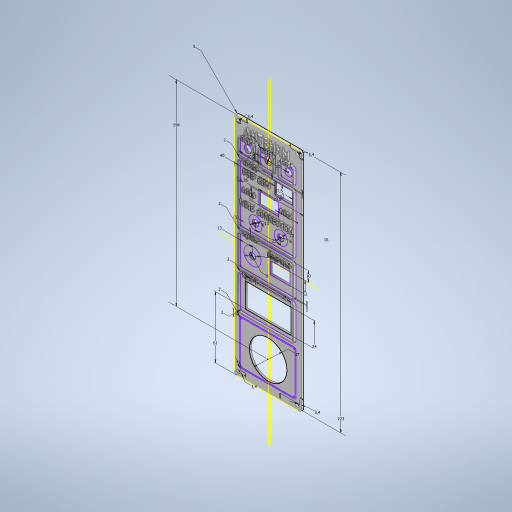
# Autodesk Inventor part: блок ЗИП и портов
Saved by Autodesk Inventor 2023.1 (Build 271208000, 208)
## iProperties
Created: 2023-03-03
Part Number: блок ЗИП и портов
Material: Типовые
Document SubType Name: Modeling
Designer: User
Density: 1 g/cm^3
Appearance: По умолчанию
Author: User
Autodesk Inventor part; units mm, degrees
(part 1 of 3)
ref_plane "YZ Plane" through (0, 0, 0) normal (1, 0, 0) x (0, 1, 0)
ref_plane "XZ Plane" through (0, 0, 0) normal (0, 1, 0) x (-1, 0, 0)
ref_plane "XY Plane" through (0, 0, 0) normal (0, 0, 1) x (1, 0, 0)
sketch "Эскиз1" plane through (0, 0, 0) normal (0, 0, 1) x (1, 0, 0)
  line L0 (-30.175, 111.5) -> (30.175, 111.5)
  line L1 (33.175, 108.5) -> (33.175, -108.5)
  line L2 (30.175, -111.5) -> (-30.175, -111.5)
  line L3 (-33.175, -108.5) -> (-33.175, 108.5)
  line L4 (0, -156.9698) -> (0, 156.9698) projected
  line L5 (-47.3148, 0) -> (47.3148, 0) projected
  arc A0 (-30.175, 111.5) -> (-33.175, 108.5) centre (-30.175, 108.5) ccw
  arc A1 (33.175, 108.5) -> (30.175, 111.5) centre (30.175, 108.5) ccw
  arc A2 (-33.175, -108.5) -> (-30.175, -111.5) centre (-30.175, -108.5) ccw
  arc A3 (30.175, -111.5) -> (33.175, -108.5) centre (30.175, -108.5) ccw
  circle A4 centre (-29.175, 107.5) radius 1.7
  circle A5 centre (29.175, 107.5) radius 1.7
  circle A6 centre (-29.175, -107.5) radius 1.7
  circle A7 centre (29.175, -107.5) radius 1.7
  point P0 (0, 0)
  dimension "d0" = 223
  dimension "d1" = 66.35
  dimension "d2" = 3
  dimension "d3" = 3.4
  dimension "d4" = 3.4
  dimension "d5" = 3.4
  dimension "d6" = 3.4
  dimension "d7" = 4
  dimension "d8" = 4
  dimension "d9" = 4
  dimension "d10" = 4
  dimension "d11" = 4
  dimension "d12" = 4
  dimension "d13" = 4
  dimension "d14" = 4
  constraints: 8 centre point, 8 end point, 8 point on circle, 8 tangent, 3 equal radius, 2 parallel, 1 horizontal, 1 perpendicular, 2 other
  measures "d0" distance between parallel lines of L2 L0
  measures "d1" distance between parallel lines of L3 L1
  measures "d2" radius of A0
  measures "d3" diameter of A4
  measures "d4" diameter of A5
  measures "d5" diameter of A6
  measures "d6" diameter of A7
  measures "d7" distance from line of L3 A6.centre
  measures "d8" distance from line of L2 A6.centre
  measures "d9" distance from line of L2 A7.centre
  measures "d10" distance from line of L1 A7.centre
  measures "d11" distance from line of A4.centre L0
  measures "d12" distance from line of L3 A4.centre
  measures "d13" distance from line of L0 A5.centre
  measures "d14" distance from line of L1 A5.centre
extrude "Выдавливание1" add sketch "Эскиз1" along normal blind 2
sketch "Эскиз2" plane through (0, 0, 2) normal (0, 0, 1) x (1, 0, 0)
  line L0 (-23.4853, 106.5513) -> (31.3754, 106.5513) construction
  line L1 (31.3754, 106.5513) -> (31.3754, 99.1453) construction
  line L2 (31.3754, 99.1453) -> (-23.4853, 99.1453) construction
  line L3 (-23.4853, 99.1453) -> (-23.4853, 106.5513) construction
  circle A0 centre (0, 87.4719) radius 3.5
  line L4 (6.5101, 93.4723) -> (6.5101, 81.4719)
  line L5 (5.5101, 80.4719) -> (-6.4899, 80.4719)
  line L6 (-7.4899, 81.4719) -> (-7.4899, 93.4723)
  arc A1 (-6.4899, 94.4723) -> (-7.4899, 93.4723) centre (-6.4899, 93.4723) ccw
  arc A2 (6.5101, 93.4723) -> (5.5101, 94.4723) centre (5.5101, 93.4723) ccw
  arc A3 (5.5101, 80.4719) -> (6.5101, 81.4719) centre (5.5101, 81.4719) ccw
  arc A4 (-7.4899, 81.4719) -> (-6.4899, 80.4719) centre (-6.4899, 81.4719) ccw
  line L7 (-8.4899, 93.4723) -> (-8.4899, 81.4719)
  arc A5 (-8.4899, 81.4719) -> (-6.4899, 79.4719) centre (-6.4899, 81.4719) ccw
  line L8 (-6.4899, 79.4719) -> (5.5101, 79.4719)
  arc A6 (5.5101, 79.4719) -> (7.5101, 81.4719) centre (5.5101, 81.4719) ccw
  line L9 (7.5101, 81.4719) -> (7.5101, 93.4723)
  arc A7 (7.5101, 93.4723) -> (5.5101, 95.4723) centre (5.5101, 93.4723) ccw
  arc A8 (-6.4899, 95.4723) -> (-8.4899, 93.4723) centre (-6.4899, 93.4723) ccw
  line L10 (-6.4899, 94.4723) -> (-6.4899, 95.4723)
  line L11 (-5.4694, 97.1945) -> (11.2685, 97.1945) construction
  line L12 (11.2685, 97.1945) -> (11.2685, 90.8671) construction
  line L13 (11.2685, 90.8671) -> (-5.4694, 90.8671) construction
  line L14 (-5.4694, 90.8671) -> (-5.4694, 97.1945) construction
  line L15 (5.5101, 94.4723) -> (5.5101, 95.4723)
  circle A9 centre (20, 87.4719) radius 3.5
  line L16 (26.5101, 93.4723) -> (26.5101, 81.4719)
  line L17 (25.5101, 80.4719) -> (13.5101, 80.4719)
  line L18 (13.5101, 79.4719) -> (25.5101, 79.4719)
  arc A10 (26.5101, 93.4723) -> (25.5101, 94.4723) centre (25.5101, 93.4723) ccw
  line L19 (27.5101, 81.4719) -> (27.5101, 93.4723)
  line L20 (25.5101, 94.4723) -> (25.5101, 95.4723)
  arc A11 (27.5101, 93.4723) -> (25.5101, 95.4723) centre (25.5101, 93.4723) ccw
  arc A12 (25.5101, 80.4719) -> (26.5101, 81.4719) centre (25.5101, 81.4719) ccw
  arc A13 (25.5101, 79.4719) -> (27.5101, 81.4719) centre (25.5101, 81.4719) ccw
  arc A14 (13.5101, 94.4723) -> (12.5101, 93.4723) centre (13.5101, 93.4723) ccw
  line L21 (13.5101, 94.4723) -> (13.5101, 95.4723)
  arc A15 (13.5101, 95.4723) -> (11.5101, 93.4723) centre (13.5101, 93.4723) ccw
  arc A16 (11.5101, 81.4719) -> (13.5101, 79.4719) centre (13.5101, 81.4719) ccw
  line L22 (12.5101, 81.4719) -> (12.5101, 93.4723)
  line L23 (11.5101, 93.4723) -> (11.5101, 81.4719)
  arc A17 (12.5101, 81.4719) -> (13.5101, 80.4719) centre (13.5101, 81.4719) ccw
  line L24 (13.4684, 97.2035) -> (30.2064, 97.2035) construction
  line L25 (30.2064, 97.2035) -> (30.2064, 90.8761) construction
  line L26 (30.2064, 90.8761) -> (13.4684, 90.8761) construction
  line L27 (13.4684, 90.8761) -> (13.4684, 97.2035) construction
  arc A18 (-28.4899, 81.4719) -> (-26.4899, 79.4719) centre (-26.4899, 81.4719) ccw
  line L28 (-12.4899, 81.4719) -> (-12.4899, 93.4723)
  arc A19 (-27.4899, 81.4719) -> (-26.4899, 80.4719) centre (-26.4899, 81.4719) ccw
  line L29 (-26.4899, 79.4719) -> (-14.4899, 79.4719)
  line L30 (-27.4899, 81.4719) -> (-27.4899, 93.4723)
  line L31 (-28.4899, 93.4723) -> (-28.4899, 81.4719)
  arc A20 (-26.4899, 95.4723) -> (-28.4899, 93.4723) centre (-26.4899, 93.4723) ccw
  arc A21 (-26.4899, 94.4723) -> (-27.4899, 93.4723) centre (-26.4899, 93.4723) ccw
  line L32 (-14.4899, 80.4719) -> (-26.4899, 80.4719)
  arc A22 (-14.4899, 80.4719) -> (-13.4899, 81.4719) centre (-14.4899, 81.4719) ccw
  line L33 (-26.4899, 94.4723) -> (-26.4899, 95.4723)
  circle A23 centre (-20, 87.4719) radius 3.5
  line L34 (-13.4899, 93.4723) -> (-13.4899, 81.4719)
  arc A24 (-13.4899, 93.4723) -> (-14.4899, 94.4723) centre (-14.4899, 93.4723) ccw
  line L35 (-14.4899, 94.4723) -> (-14.4899, 95.4723)
  arc A25 (-12.4899, 93.4723) -> (-14.4899, 95.4723) centre (-14.4899, 93.4723) ccw
  arc A26 (-14.4899, 79.4719) -> (-12.4899, 81.4719) centre (-14.4899, 81.4719) ccw
  line L36 (-25.5636, 97.0542) -> (-8.8256, 97.0542) construction
  line L37 (-8.8256, 97.0542) -> (-8.8256, 90.7268) construction
  line L38 (-8.8256, 90.7268) -> (-25.5636, 90.7268) construction
  line L39 (-25.5636, 90.7268) -> (-25.5636, 97.0542) construction
  line L40 (6.825, 73.4719) -> (24.325, 73.4719)
  line L41 (24.325, 73.4719) -> (24.325, 61.4719)
  line L42 (24.325, 61.4719) -> (6.825, 61.4719)
  line L43 (6.825, 61.4719) -> (6.825, 73.4719)
  line L44 (0, -156.1) -> (0, 156.1) projected
  line L45 (-23.9479, 69.9979) -> (9.951, 69.9979) construction
  line L46 (9.951, 69.9979) -> (9.951, 63.8878) construction
  line L47 (9.951, 63.8878) -> (-23.9479, 63.8878) construction
  line L48 (-23.9479, 63.8878) -> (-23.9479, 69.9979) construction
  line L49 (-33.175, 108.5) -> (-33.175, -108.5) projected
  line L50 (27.5101, 74.3869) -> (27.5101, 19.3056)
  line L51 (25.5101, 17.3056) -> (-26.4899, 17.3056)
  line L52 (-28.4899, 19.3056) -> (-28.4899, 74.3869)
  arc A27 (-26.4899, 76.3869) -> (-28.4899, 74.3869) centre (-26.4899, 74.3869) ccw
  arc A28 (27.5101, 74.3869) -> (25.5101, 76.3869) centre (25.5101, 74.3869) ccw
  arc A29 (25.5101, 17.3056) -> (27.5101, 19.3056) centre (25.5101, 19.3056) ccw
  arc A30 (-28.4899, 19.3056) -> (-26.4899, 17.3056) centre (-26.4899, 19.3056) ccw
  arc A31 (-26.4899, 75.3869) -> (-27.4899, 74.3869) centre (-26.4899, 74.3869) ccw
  line L53 (-27.4899, 74.3869) -> (-27.4899, 19.3056)
  arc A32 (-27.4899, 19.3056) -> (-26.4899, 18.3056) centre (-26.4899, 19.3056) ccw
  line L54 (-26.4899, 18.3056) -> (25.5101, 18.3056)
  arc A33 (25.5101, 18.3056) -> (26.5101, 19.3056) centre (25.5101, 19.3056) ccw
  line L55 (26.5101, 19.3056) -> (26.5101, 74.3869)
  arc A34 (26.5101, 74.3869) -> (25.5101, 75.3869) centre (25.5101, 74.3869) ccw
  line L56 (-24.4499, 53.724) -> (9.4489, 53.724) construction
  line L57 (9.4489, 53.724) -> (9.4489, 47.6139) construction
  line L58 (9.4489, 47.6139) -> (-24.4499, 47.6139) construction
  line L59 (-24.4499, 47.6139) -> (-24.4499, 53.724) construction
  line L60 (-8.9899, 57.0024) -> (10.5101, 57.0024)
  line L61 (10.5101, 57.0024) -> (10.5101, 45.0024)
  line L62 (10.5101, 45.0024) -> (-8.9899, 45.0024)
  line L63 (-8.9899, 45.0024) -> (-8.9899, 57.0024)
  line L64 (12.474, 47.646) -> (12.474, 53.7562) construction
  line L65 (12.474, 53.7562) -> (46.3728, 53.7562) construction
  line L66 (46.3728, 53.7562) -> (46.3728, 47.646) construction
  line L67 (46.3728, 47.646) -> (12.474, 47.646) construction
  line L68 (-27.2571, 42.4637) -> (29.1197, 42.4637) construction
  line L69 (29.1197, 42.4637) -> (29.1197, 45.205) construction
  line L70 (29.1197, 45.205) -> (-27.2571, 45.205) construction
  line L71 (-27.2571, 45.205) -> (-27.2571, 42.4637) construction
  circle A35 centre (-12.5, 27.8557) radius 3
  circle A36 centre (12.5, 27.8557) radius 3
  circle A37 centre (-12.5, 27.8557) radius 6.5
  circle A38 centre (12.5, 27.8557) radius 6.5
  line L72 (-24.9853, 76.3869) -> (-24.9853, 75.3869)
  line L73 (-26.4899, 76.3869) -> (-24.9853, 76.3869)
  line L74 (-6.4899, 76.3869) -> (25.5101, 76.3869)
  line L75 (-24.9853, 75.3869) -> (-26.4899, 75.3869)
  line L76 (-23.3758, 71.3083) -> (-23.3758, 77.6357) construction
  line L77 (-23.3758, 77.6357) -> (-6.6378, 77.6357) construction
  line L78 (-6.6378, 77.6357) -> (-6.6378, 71.3083) construction
  line L79 (-6.6378, 71.3083) -> (-23.3758, 71.3083) construction
  line L80 (-6.4899, 76.3869) -> (-6.4899, 75.3869)
  line L81 (25.5101, 75.3869) -> (-6.4899, 75.3869)
  line L82 (-12.4899, 74.9766) -> (-12.5, 74.9766)
  line L83 (27.5101, 12.3056) -> (27.5101, -15.7398)
  line L84 (25.5101, -17.7398) -> (-26.4899, -17.7398)
  line L85 (-28.4899, -15.7398) -> (-28.4899, 12.3056)
  arc A39 (-26.4899, 14.3056) -> (-28.4899, 12.3056) centre (-26.4899, 12.3056) ccw
  arc A40 (-28.4899, -15.7398) -> (-26.4899, -17.7398) centre (-26.4899, -15.7398) ccw
  arc A41 (25.5101, -17.7398) -> (27.5101, -15.7398) centre (25.5101, -15.7398) ccw
  arc A42 (27.5101, 12.3056) -> (25.5101, 14.3056) centre (25.5101, 12.3056) ccw
  arc A43 (-26.4899, 13.3056) -> (-27.4899, 12.3056) centre (-26.4899, 12.3056) ccw
  line L86 (-27.4899, 12.3056) -> (-27.4899, -15.7398)
  arc A44 (-27.4899, -15.7398) -> (-26.4899, -16.7398) centre (-26.4899, -15.7398) ccw
  line L87 (-26.4899, -16.7398) -> (25.5101, -16.7398)
  arc A45 (25.5101, -16.7398) -> (26.5101, -15.7398) centre (25.5101, -15.7398) ccw
  line L88 (26.5101, -15.7398) -> (26.5101, 12.3056)
  arc A46 (26.5101, 12.3056) -> (25.5101, 13.3056) centre (25.5101, 12.3056) ccw
  line L89 (-24.4499, 14.3056) -> (-24.4499, 13.3056)
  line L90 (-26.4899, 14.3056) -> (-24.4499, 14.3056)
  line L91 (-8.4899, 14.3056) -> (25.5101, 14.3056)
  line L92 (25.5101, 13.3056) -> (-8.4899, 13.3056)
  line L93 (-24.4499, 13.3056) -> (-26.4899, 13.3056)
  line L94 (-23.3782, 9.1957) -> (-23.3782, 15.5231) construction
  line L95 (-23.3782, 15.5231) -> (-6.6403, 15.5231) construction
  line L96 (-6.6403, 15.5231) -> (-6.6403, 9.1957) construction
  line L97 (-6.6403, 9.1957) -> (-23.3782, 9.1957) construction
  line L98 (-8.4899, 14.3056) -> (-8.4899, 13.3056)
  circle A47 centre (-15.4899, -1.7171) radius 3
  circle A48 centre (-15.4899, -1.7171) radius 8.5
  line L99 (2.2026, 3.3056) -> (21.7026, 3.3056)
  line L100 (21.7026, 3.3056) -> (21.7026, -8.6944)
  line L101 (21.7026, -8.6944) -> (2.2026, -8.6944)
  line L102 (2.2026, -8.6944) -> (2.2026, 3.3056)
  line L103 (0.6713, 5.0746) -> (0.6713, 11.009) construction
  line L104 (0.6713, 11.009) -> (17.4092, 11.009) construction
  line L105 (17.4092, 11.009) -> (17.4092, 5.0746) construction
  line L106 (17.4092, 5.0746) -> (0.6713, 5.0746) construction
  line L107 (27.5101, -22.4503) -> (27.5101, -52.9823)
  line L108 (25.5101, -54.9823) -> (-26.4899, -54.9823)
  line L109 (-28.4899, -52.9823) -> (-28.4899, -22.4503)
  arc A49 (-26.4899, -20.4503) -> (-28.4899, -22.4503) centre (-26.4899, -22.4503) ccw
  arc A50 (-28.4899, -52.9823) -> (-26.4899, -54.9823) centre (-26.4899, -52.9823) ccw
  arc A51 (25.5101, -54.9823) -> (27.5101, -52.9823) centre (25.5101, -52.9823) ccw
  arc A52 (27.5101, -22.4503) -> (25.5101, -20.4503) centre (25.5101, -22.4503) ccw
  arc A53 (-26.4899, -21.4503) -> (-27.4899, -22.4503) centre (-26.4899, -22.4503) ccw
  line L110 (-27.4899, -22.4503) -> (-27.4899, -52.9823)
  arc A54 (-27.4899, -52.9823) -> (-26.4899, -53.9823) centre (-26.4899, -52.9823) ccw
  line L111 (-26.4899, -53.9823) -> (25.5101, -53.9823)
  arc A55 (25.5101, -53.9823) -> (26.5101, -52.9823) centre (25.5101, -52.9823) ccw
  line L112 (26.5101, -52.9823) -> (26.5101, -22.4503)
  arc A56 (26.5101, -22.4503) -> (25.5101, -21.4503) centre (25.5101, -22.4503) ccw
  line L113 (-22.5, -26.5) -> (22.5, -26.5)
  line L114 (22.5, -26.5) -> (22.5, -50.5)
  line L115 (22.5, -50.5) -> (-22.5, -50.5)
  line L116 (-22.5, -50.5) -> (-22.5, -26.5)
  line L117 (-30.175, -111.5) -> (30.175, -111.5) projected
  line L118 (-25.4699, -20.4503) -> (-25.4699, -21.4503)
  line L119 (-8.4899, -20.4503) -> (-8.4899, -21.4503)
  line L120 (25.5101, -21.4503) -> (-8.4899, -21.4503)
  line L121 (-25.4699, -21.4503) -> (-26.4899, -21.4503)
  line L122 (-26.4899, -20.4503) -> (-25.4699, -20.4503)
  line L123 (-8.4899, -20.4503) -> (25.5101, -20.4503)
  line L124 (-23.7978, -25.6666) -> (-23.7978, -19.3393) construction
  line L125 (-23.7978, -19.3393) -> (-7.0599, -19.3393) construction
  line L126 (-7.0599, -19.3393) -> (-7.0599, -25.6666) construction
  line L127 (-7.0599, -25.6666) -> (-23.7978, -25.6666) construction
  circle A57 centre (0, -82.5) radius 18.5
  line L128 (30.175, 111.5) -> (-30.175, 111.5) projected
  line L129 (-26.4899, -58.9749) -> (25.5101, -58.9749)
  line L130 (27.5101, -60.9749) -> (27.5101, -101.3327)
  line L131 (25.5101, -103.3327) -> (-26.4899, -103.3327)
  line L132 (-28.4899, -101.3327) -> (-28.4899, -60.9749)
  arc A58 (-26.4899, -58.9749) -> (-28.4899, -60.9749) centre (-26.4899, -60.9749) ccw
  arc A59 (27.5101, -60.9749) -> (25.5101, -58.9749) centre (25.5101, -60.9749) ccw
  arc A60 (25.5101, -103.3327) -> (27.5101, -101.3327) centre (25.5101, -101.3327) ccw
  arc A61 (-28.4899, -101.3327) -> (-26.4899, -103.3327) centre (-26.4899, -101.3327) ccw
  line L133 (25.5101, -59.9749) -> (-26.4899, -59.9749)
  arc A62 (-26.4899, -59.9749) -> (-27.4899, -60.9749) centre (-26.4899, -60.9749) ccw
  line L134 (-27.4899, -60.9749) -> (-27.4899, -101.3327)
  arc A63 (-27.4899, -101.3327) -> (-26.4899, -102.3327) centre (-26.4899, -101.3327) ccw
  line L135 (-26.4899, -102.3327) -> (25.5101, -102.3327)
  arc A64 (25.5101, -102.3327) -> (26.5101, -101.3327) centre (25.5101, -101.3327) ccw
  line L136 (26.5101, -101.3327) -> (26.5101, -60.9749)
  arc A65 (26.5101, -60.9749) -> (25.5101, -59.9749) centre (25.5101, -60.9749) ccw
  line L137 (-23.2368, 95.4767) -> (-23.2368, 96.7836)
  spline S0 degree 2 poles (-23.2368, 96.7836) (-23.2368, 97.0344) (-22.986, 97.0344) knots 0 0 0 1 1 1
  spline S1 degree 2 poles (-22.986, 97.0344) (-22.7352, 97.0344) (-22.7352, 96.7836) knots 0 0 0 1 1 1
  line L138 (-22.7352, 96.7836) -> (-22.7352, 93.2985)
  spline S2 degree 2 poles (-22.7352, 93.2985) (-22.7352, 93.0443) (-22.9926, 93.0443) knots 0 0 0 1 1 1
  spline S3 degree 2 poles (-22.9926, 93.0443) (-23.2368, 93.0443) (-23.2368, 93.2919) knots 0 0 0 1 1 1
  line L139 (-23.2368, 93.2919) -> (-23.2368, 94.9783)
  line L140 (-23.2368, 94.9783) -> (-24.6758, 94.9783)
  line L141 (-24.6758, 94.9783) -> (-24.6758, 93.2919)
  spline S4 degree 2 poles (-24.6758, 93.2919) (-24.6758, 93.041) (-24.9266, 93.041) knots 0 0 0 1 1 1
  spline S5 degree 2 poles (-24.9266, 93.041) (-25.1774, 93.041) (-25.1774, 93.2919) knots 0 0 0 1 1 1
  line L142 (-25.1774, 93.2919) -> (-25.1774, 96.777)
  spline S6 degree 2 poles (-25.1774, 96.777) (-25.1774, 97.0278) (-24.9266, 97.0278) knots 0 0 0 1 1 1
  spline S7 degree 2 poles (-24.9266, 97.0278) (-24.6758, 97.0278) (-24.6758, 96.777) knots 0 0 0 1 1 1
  line L143 (-24.6758, 96.777) -> (-24.6758, 95.4767)
  line L144 (-24.6758, 95.4767) -> (-23.2368, 95.4767)
  line L145 (-20.2731, 93.041) -> (-21.0487, 93.041)
  spline S8 degree 2 poles (-21.0487, 93.041) (-21.4745, 93.041) (-22.0718, 93.6384) (-22.0718, 94.0674) knots 0 0 0 1 2 2 2
  line L146 (-22.0718, 94.0674) -> (-22.0718, 96.0047)
  spline S9 degree 2 poles (-22.0718, 96.0047) (-22.0718, 96.4305) (-21.4745, 97.0278) (-21.0487, 97.0278) knots 0 0 0 1 2 2 2
  line L147 (-21.0487, 97.0278) -> (-20.2731, 97.0278)
  spline S10 degree 2 poles (-20.2731, 97.0278) (-20.019, 97.0278) (-20.019, 96.7803) knots 0 0 0 1 1 1
  spline S11 degree 2 poles (-20.019, 96.7803) (-20.019, 96.5295) (-20.2731, 96.5295) knots 0 0 0 1 1 1
  line L148 (-20.2731, 96.5295) -> (-21.0487, 96.5295)
  spline S12 degree 2 poles (-21.0487, 96.5295) (-21.2632, 96.5295) (-21.5702, 96.2226) (-21.5702, 96.0047) knots 0 0 0 1 2 2 2
  line L149 (-21.5702, 96.0047) -> (-21.5702, 94.0641)
  spline S13 degree 2 poles (-21.5702, 94.0641) (-21.5702, 93.8463) (-21.2632, 93.5394) (-21.0487, 93.5394) knots 0 0 0 1 2 2 2
  line L150 (-21.0487, 93.5394) -> (-20.2731, 93.5394)
  spline S14 degree 2 poles (-20.2731, 93.5394) (-20.019, 93.5394) (-20.019, 93.2919) knots 0 0 0 1 1 1
  spline S15 degree 2 poles (-20.019, 93.2919) (-20.019, 93.041) (-20.2731, 93.041) knots 0 0 0 1 1 1
  spline S16 degree 2 poles (-18.0817, 93.2919) (-18.0817, 93.041) (-18.3325, 93.041) knots 0 0 0 1 1 1
  spline S17 degree 2 poles (-18.3325, 93.041) (-18.5834, 93.041) (-18.5834, 93.2886) knots 0 0 0 1 1 1
  line L151 (-18.5834, 93.2886) -> (-18.5834, 96.2556)
  line L152 (-18.5834, 96.2556) -> (-18.9332, 95.8265)
  spline S18 degree 2 poles (-18.9332, 95.8265) (-19.0058, 95.7539) (-19.1048, 95.7539) knots 0 0 0 1 1 1
  spline S19 degree 2 poles (-19.1048, 95.7539) (-19.2071, 95.7539) (-19.3589, 95.9057) (-19.3589, 96.008) knots 0 0 0 1 2 2 2
  spline S20 degree 2 poles (-19.3589, 96.008) (-19.3589, 96.1037) (-19.2863, 96.1763) knots 0 0 0 1 1 1
  line L153 (-19.2863, 96.1763) -> (-18.5108, 96.9519)
  spline S21 degree 2 poles (-18.5108, 96.9519) (-18.4084, 97.0542) (-18.2995, 97.0542) knots 0 0 0 1 1 1
  spline S22 degree 2 poles (-18.2995, 97.0542) (-18.0817, 97.0542) (-18.0817, 96.777) knots 0 0 0 1 1 1
  line L154 (-18.0817, 96.777) -> (-18.0817, 93.2919)
  line L155 (-15.5075, 95.4833) -> (-16.7616, 93.5394)
  line L156 (-16.7616, 93.5394) -> (-15.6197, 93.5394)
  spline S23 degree 2 poles (-15.6197, 93.5394) (-15.3655, 93.5394) (-15.3655, 93.2919) knots 0 0 0 1 1 1
  spline S24 degree 2 poles (-15.3655, 93.2919) (-15.3655, 93.041) (-15.6197, 93.041) knots 0 0 0 1 1 1
  line L157 (-15.6197, 93.041) -> (-17.1708, 93.041)
  spline S25 degree 2 poles (-17.1708, 93.041) (-17.4348, 93.041) (-17.4348, 93.2523) knots 0 0 0 1 1 1
  spline S26 degree 2 poles (-17.4348, 93.2523) (-17.4348, 93.3315) (-17.3688, 93.4437) knots 0 0 0 1 1 1
  line L158 (-17.3688, 93.4437) -> (-15.9497, 95.7044)
  spline S27 degree 2 poles (-15.9497, 95.7044) (-15.8738, 95.8298) (-15.8738, 95.9717) knots 0 0 0 1 1 1
  spline S28 degree 2 poles (-15.8738, 95.9717) (-15.8738, 96.1895) (-16.2137, 96.5262) (-16.4579, 96.5262) knots 0 0 0 1 2 2 2
  spline S29 degree 2 poles (-16.4579, 96.5262) (-16.7814, 96.5262) (-16.9563, 96.2523) knots 0 0 0 1 1 1
  spline S30 degree 2 poles (-16.9563, 96.2523) (-17.0322, 96.14) (-17.1609, 96.14) knots 0 0 0 1 1 1
  spline S31 degree 2 poles (-17.1609, 96.14) (-17.2665, 96.14) (-17.4249, 96.282) (-17.4249, 96.3876) knots 0 0 0 1 2 2 2
  spline S32 degree 2 poles (-17.4249, 96.3876) (-17.4249, 96.4602) (-17.3754, 96.5328) knots 0 0 0 1 1 1
  spline S33 degree 2 poles (-17.3754, 96.5328) (-17.0487, 97.0311) (-16.4579, 97.0311) knots 0 0 0 1 1 1
  spline S34 degree 2 poles (-16.4579, 97.0311) (-16.0058, 97.0311) (-15.3655, 96.3843) (-15.3655, 95.9651) knots 0 0 0 1 2 2 2
  spline S35 degree 2 poles (-15.3655, 95.9651) (-15.3655, 95.6879) (-15.5075, 95.4833) knots 0 0 0 1 1 1
  spline S36 degree 2 poles (-20.4591, 66.2427) (-20.4591, 65.7265) (-21.1877, 64.9979) (-21.7039, 64.9979) knots 0 0 0 1 2 2 2
  line L159 (-21.7039, 64.9979) -> (-22.2035, 64.9979)
  spline S37 degree 2 poles (-22.2035, 64.9979) (-22.7197, 64.9979) (-23.4483, 65.7265) (-23.4483, 66.2427) knots 0 0 0 1 2 2 2
  line L160 (-23.4483, 66.2427) -> (-23.4483, 69.7315)
  spline S38 degree 2 poles (-23.4483, 69.7315) (-23.4483, 69.9813) (-23.1985, 69.9813) knots 0 0 0 1 1 1
  spline S39 degree 2 poles (-23.1985, 69.9813) (-22.9487, 69.9813) (-22.9487, 69.7315) knots 0 0 0 1 1 1
  line L161 (-22.9487, 69.7315) -> (-22.9487, 66.2469)
  spline S40 degree 2 poles (-22.9487, 66.2469) (-22.9487, 65.9346) (-22.5116, 65.4975) (-22.2035, 65.4975) knots 0 0 0 1 2 2 2
  line L162 (-22.2035, 65.4975) -> (-21.7039, 65.4975)
  spline S41 degree 2 poles (-21.7039, 65.4975) (-21.3958, 65.4975) (-20.9587, 65.9346) (-20.9587, 66.2469) knots 0 0 0 1 2 2 2
  line L163 (-20.9587, 66.2469) -> (-20.9587, 69.7315)
  spline S42 degree 2 poles (-20.9587, 69.7315) (-20.9587, 69.9813) (-20.7089, 69.9813) knots 0 0 0 1 1 1
  spline S43 degree 2 poles (-20.7089, 69.9813) (-20.4591, 69.9813) (-20.4591, 69.7315) knots 0 0 0 1 1 1
  line L164 (-20.4591, 69.7315) -> (-20.4591, 66.2427)
  spline S44 degree 2 poles (-16.6248, 69.5608) (-16.5124, 69.4817) (-16.5124, 69.361) knots 0 0 0 1 1 1
  spline S45 degree 2 poles (-16.5124, 69.361) (-16.5124, 69.261) (-16.6623, 69.1028) (-16.7622, 69.1028) knots 0 0 0 1 2 2 2
  spline S46 degree 2 poles (-16.7622, 69.1028) (-16.8413, 69.1028) (-16.9121, 69.1528) knots 0 0 0 1 1 1
  spline S47 degree 2 poles (-16.9121, 69.1528) (-17.3867, 69.4942) (-17.9654, 69.4942) knots 0 0 0 1 1 1
  spline S48 degree 2 poles (-17.9654, 69.4942) (-18.3401, 69.4942) (-18.9437, 69.1819) (-18.9437, 68.8822) knots 0 0 0 1 2 2 2
  spline S49 degree 2 poles (-18.9437, 68.8822) (-18.9437, 68.7032) (-18.8022, 68.5949) knots 0 0 0 1 1 1
  line L165 (-18.8022, 68.5949) -> (-16.9537, 67.2294)
  spline S50 degree 2 poles (-16.9537, 67.2294) (-16.4541, 66.863) (-16.4541, 66.2053) knots 0 0 0 1 1 1
  spline S51 degree 2 poles (-16.4541, 66.2053) (-16.4541, 65.5225) (-17.5033, 64.9729) (-18.007, 64.9729) knots 0 0 0 1 2 2 2
  spline S52 degree 2 poles (-18.007, 64.9729) (-18.6398, 64.9729) (-19.3267, 65.4184) knots 0 0 0 1 1 1
  spline S53 degree 2 poles (-19.3267, 65.4184) (-19.4433, 65.4933) (-19.4433, 65.6182) knots 0 0 0 1 1 1
  spline S54 degree 2 poles (-19.4433, 65.6182) (-19.4433, 65.7223) (-19.2976, 65.8805) (-19.1935, 65.8805) knots 0 0 0 1 2 2 2
  spline S55 degree 2 poles (-19.1935, 65.8805) (-19.1227, 65.8805) (-19.0603, 65.8347) knots 0 0 0 1 1 1
  spline S56 degree 2 poles (-19.0603, 65.8347) (-18.4941, 65.4725) (-17.9945, 65.4725) knots 0 0 0 1 1 1
  spline S57 degree 2 poles (-17.9945, 65.4725) (-17.6115, 65.4725) (-17.2077, 65.6807) knots 0 0 0 1 1 1
  spline S58 degree 2 poles (-17.2077, 65.6807) (-16.9371, 65.8264) (-16.9371, 66.1969) knots 0 0 0 1 1 1
  spline S59 degree 2 poles (-16.9371, 66.1969) (-16.9371, 66.6008) (-17.2326, 66.8172) knots 0 0 0 1 1 1
  line L166 (-17.2326, 66.8172) -> (-19.0811, 68.1869)
  spline S60 degree 2 poles (-19.0811, 68.1869) (-19.4225, 68.4367) (-19.4225, 68.8905) knots 0 0 0 1 1 1
  spline S61 degree 2 poles (-19.4225, 68.8905) (-19.4225, 69.4859) (-18.8688, 69.7773) knots 0 0 0 1 1 1
  spline S62 degree 2 poles (-18.8688, 69.7773) (-18.4691, 69.9813) (-17.9654, 69.9813) knots 0 0 0 1 1 1
  spline S63 degree 2 poles (-17.9654, 69.9813) (-17.216, 69.9813) (-16.6248, 69.5608) knots 0 0 0 1 1 1
  spline S64 degree 2 poles (-12.3575, 66.4925) (-12.3575, 65.8764) (-13.236, 64.9979) (-13.8521, 64.9979) knots 0 0 0 1 2 2 2
  line L167 (-13.8521, 64.9979) -> (-15.3467, 64.9979)
  spline S65 degree 2 poles (-15.3467, 64.9979) (-15.455, 64.9979) (-15.5965, 65.1395) (-15.5965, 65.2477) knots 0 0 0 1 2 2 2
  line L168 (-15.5965, 65.2477) -> (-15.5965, 69.7315)
  spline S66 degree 2 poles (-15.5965, 69.7315) (-15.5965, 69.8314) (-15.4466, 69.9813) (-15.3467, 69.9813) knots 0 0 0 1 2 2 2
  line L169 (-15.3467, 69.9813) -> (-13.8521, 69.9813)
  spline S67 degree 2 poles (-13.8521, 69.9813) (-13.3359, 69.9813) (-12.6073, 69.2486) (-12.6073, 68.7365) knots 0 0 0 1 2 2 2
  spline S68 degree 2 poles (-12.6073, 68.7365) (-12.6073, 68.1411) (-13.0736, 67.7665) knots 0 0 0 1 1 1
  spline S69 degree 2 poles (-13.0736, 67.7665) (-12.3575, 67.3252) (-12.3575, 66.4925) knots 0 0 0 1 1 1
  spline S70 degree 2 poles (-12.8571, 66.4925) (-12.8571, 66.9047) (-13.44, 67.4875) (-13.8521, 67.4875) knots 0 0 0 1 2 2 2
  line L170 (-13.8521, 67.4875) -> (-15.0969, 67.4875)
  line L171 (-15.0969, 67.4875) -> (-15.0969, 65.4975)
  line L172 (-15.0969, 65.4975) -> (-13.8521, 65.4975)
  spline S71 degree 2 poles (-13.8521, 65.4975) (-13.44, 65.4975) (-12.8571, 66.0804) (-12.8571, 66.4925) knots 0 0 0 1 2 2 2
  spline S72 degree 2 poles (-13.1069, 68.7365) (-13.1069, 69.0446) (-13.544, 69.4817) (-13.8521, 69.4817) knots 0 0 0 1 2 2 2
  line L173 (-13.8521, 69.4817) -> (-15.0969, 69.4817)
  line L174 (-15.0969, 69.4817) -> (-15.0969, 67.9871)
  line L175 (-15.0969, 67.9871) -> (-13.8521, 67.9871)
  spline S73 degree 2 poles (-13.8521, 67.9871) (-13.544, 67.9871) (-13.1069, 68.4242) (-13.1069, 68.7365) knots 0 0 0 1 2 2 2
  line L176 (-6.2501, 64.9979) -> (-7.2451, 64.9979)
  spline S74 degree 2 poles (-7.2451, 64.9979) (-7.7655, 64.9979) (-8.4941, 65.7265) (-8.4941, 66.2427) knots 0 0 0 1 2 2 2
  line L177 (-8.4941, 66.2427) -> (-8.4941, 68.7365)
  spline S75 degree 2 poles (-8.4941, 68.7365) (-8.4941, 69.2527) (-7.7655, 69.9813) (-7.2451, 69.9813) knots 0 0 0 1 2 2 2
  line L178 (-7.2451, 69.9813) -> (-6.2501, 69.9813)
  spline S76 degree 2 poles (-6.2501, 69.9813) (-6.0003, 69.9813) (-6.0003, 69.7315) knots 0 0 0 1 1 1
  spline S77 degree 2 poles (-6.0003, 69.7315) (-6.0003, 69.4817) (-6.2501, 69.4817) knots 0 0 0 1 1 1
  line L179 (-6.2501, 69.4817) -> (-7.2451, 69.4817)
  spline S78 degree 2 poles (-7.2451, 69.4817) (-7.5574, 69.4817) (-7.9945, 69.0446) (-7.9945, 68.7365) knots 0 0 0 1 2 2 2
  line L180 (-7.9945, 68.7365) -> (-7.9945, 66.2427)
  spline S79 degree 2 poles (-7.9945, 66.2427) (-7.9945, 65.9346) (-7.5574, 65.4975) (-7.2451, 65.4975) knots 0 0 0 1 2 2 2
  line L181 (-7.2451, 65.4975) -> (-6.2501, 65.4975)
  spline S80 degree 2 poles (-6.2501, 65.4975) (-6.0003, 65.4975) (-6.0003, 65.2477) knots 0 0 0 1 1 1
  spline S81 degree 2 poles (-6.0003, 65.2477) (-6.0003, 64.9979) (-6.2501, 64.9979) knots 0 0 0 1 1 1
  spline S82 degree 2 poles (-2.0162, 66.2427) (-2.0162, 65.7265) (-2.7447, 64.9979) (-3.261, 64.9979) knots 0 0 0 1 2 2 2
  line L182 (-3.261, 64.9979) -> (-3.7605, 64.9979)
  spline S83 degree 2 poles (-3.7605, 64.9979) (-4.2768, 64.9979) (-5.0053, 65.7265) (-5.0053, 66.2427) knots 0 0 0 1 2 2 2
  line L183 (-5.0053, 66.2427) -> (-5.0053, 68.7365)
  spline S84 degree 2 poles (-5.0053, 68.7365) (-5.0053, 69.2486) (-4.2768, 69.9813) (-3.7605, 69.9813) knots 0 0 0 1 2 2 2
  line L184 (-3.7605, 69.9813) -> (-3.261, 69.9813)
  spline S85 degree 2 poles (-3.261, 69.9813) (-2.7447, 69.9813) (-2.0162, 69.2486) (-2.0162, 68.7365) knots 0 0 0 1 2 2 2
  line L185 (-2.0162, 68.7365) -> (-2.0162, 66.2427)
  line L186 (-2.5157, 66.2427) -> (-2.5157, 68.7365)
  spline S86 degree 2 poles (-2.5157, 68.7365) (-2.5157, 69.0446) (-2.9529, 69.4817) (-3.261, 69.4817) knots 0 0 0 1 2 2 2
  line L187 (-3.261, 69.4817) -> (-3.7605, 69.4817)
  spline S87 degree 2 poles (-3.7605, 69.4817) (-4.0686, 69.4817) (-4.5057, 69.0446) (-4.5057, 68.7365) knots 0 0 0 1 2 2 2
  line L188 (-4.5057, 68.7365) -> (-4.5057, 66.2427)
  spline S88 degree 2 poles (-4.5057, 66.2427) (-4.5057, 65.9346) (-4.0686, 65.4975) (-3.7605, 65.4975) knots 0 0 0 1 2 2 2
  line L189 (-3.7605, 65.4975) -> (-3.261, 65.4975)
  spline S89 degree 2 poles (-3.261, 65.4975) (-2.9529, 65.4975) (-2.5157, 65.9346) (-2.5157, 66.2427) knots 0 0 0 1 2 2 2
  spline S90 degree 2 poles (2.4759, 65.2477) (2.4759, 64.9979) (2.2261, 64.9979) knots 0 0 0 1 1 1
  spline S91 degree 2 poles (2.2261, 64.9979) (1.9764, 64.9979) (1.9764, 65.2477) knots 0 0 0 1 1 1
  line L190 (1.9764, 65.2477) -> (1.9764, 68.8073)
  line L191 (1.9764, 68.8073) -> (0.948, 67.0837)
  spline S92 degree 2 poles (0.948, 67.0837) (0.8523, 66.9255) (0.7316, 66.9255) knots 0 0 0 1 1 1
  spline S93 degree 2 poles (0.7316, 66.9255) (0.6108, 66.9255) (0.5192, 67.0837) knots 0 0 0 1 1 1
  line L192 (0.5192, 67.0837) -> (-0.5174, 68.8073)
  line L193 (-0.5174, 68.8073) -> (-0.5174, 65.2477)
  spline S94 degree 2 poles (-0.5174, 65.2477) (-0.5174, 64.9979) (-0.7672, 64.9979) knots 0 0 0 1 1 1
  spline S95 degree 2 poles (-0.7672, 64.9979) (-1.017, 64.9979) (-1.017, 65.2477) knots 0 0 0 1 1 1
  line L194 (-1.017, 65.2477) -> (-1.017, 69.7107)
  spline S96 degree 2 poles (-1.017, 69.7107) (-1.017, 69.9979) (-0.7922, 69.9979) knots 0 0 0 1 1 1
  spline S97 degree 2 poles (-0.7922, 69.9979) (-0.6465, 69.9979) (-0.5507, 69.8397) knots 0 0 0 1 1 1
  line L195 (-0.5507, 69.8397) -> (0.7316, 67.6998)
  line L196 (0.7316, 67.6998) -> (2.0097, 69.8397)
  spline S98 degree 2 poles (2.0097, 69.8397) (2.1054, 69.9979) (2.247, 69.9979) knots 0 0 0 1 1 1
  spline S99 degree 2 poles (2.247, 69.9979) (2.4759, 69.9979) (2.4759, 69.7107) knots 0 0 0 1 1 1
  line L197 (2.4759, 69.7107) -> (2.4759, 65.2477)
  spline S100 degree 2 poles (-2.641, 93.4453) (-2.641, 93.343) (-2.7895, 93.1945) (-2.8952, 93.1945) knots 0 0 0 1 2 2 2
  line L198 (-2.8952, 93.1945) -> (-4.0569, 93.1945)
  spline S101 degree 2 poles (-4.0569, 93.1945) (-4.4826, 93.1945) (-5.08, 93.7918) (-5.08, 94.2209) knots 0 0 0 1 2 2 2
  line L199 (-5.08, 94.2209) -> (-5.08, 96.1582)
  spline S102 degree 2 poles (-5.08, 96.1582) (-5.08, 96.5839) (-4.4826, 97.1813) (-4.0569, 97.1813) knots 0 0 0 1 2 2 2
  line L200 (-4.0569, 97.1813) -> (-2.8952, 97.1813)
  spline S103 degree 2 poles (-2.8952, 97.1813) (-2.641, 97.1813) (-2.641, 96.9337) knots 0 0 0 1 1 1
  spline S104 degree 2 poles (-2.641, 96.9337) (-2.641, 96.6829) (-2.8952, 96.6829) knots 0 0 0 1 1 1
  line L201 (-2.8952, 96.6829) -> (-4.0569, 96.6829)
  spline S105 degree 2 poles (-4.0569, 96.6829) (-4.2714, 96.6829) (-4.5783, 96.376) (-4.5783, 96.1582) knots 0 0 0 1 2 2 2
  line L202 (-4.5783, 96.1582) -> (-4.5783, 94.2176)
  spline S106 degree 2 poles (-4.5783, 94.2176) (-4.5783, 93.9997) (-4.2714, 93.6928) (-4.0569, 93.6928) knots 0 0 0 1 2 2 2
  line L203 (-4.0569, 93.6928) -> (-3.1427, 93.6928)
  line L204 (-3.1427, 93.6928) -> (-3.1427, 95.1318)
  line L205 (-3.1427, 95.1318) -> (-3.2813, 95.1318)
  spline S107 degree 2 poles (-3.2813, 95.1318) (-3.5321, 95.1318) (-3.5321, 95.3826) knots 0 0 0 1 1 1
  spline S108 degree 2 poles (-3.5321, 95.3826) (-3.5321, 95.6301) (-3.2813, 95.6301) knots 0 0 0 1 1 1
  line L206 (-3.2813, 95.6301) -> (-2.8952, 95.6301)
  spline S109 degree 2 poles (-2.8952, 95.6301) (-2.7928, 95.6301) (-2.641, 95.4783) (-2.641, 95.3793) knots 0 0 0 1 2 2 2
  line L207 (-2.641, 95.3793) -> (-2.641, 93.4453)
  spline S110 degree 2 poles (0.3029, 96.8512) (0.425, 96.7621) (0.425, 96.6433) knots 0 0 0 1 1 1
  spline S111 degree 2 poles (0.425, 96.6433) (0.425, 96.5443) (0.2765, 96.3859) (0.1709, 96.3859) knots 0 0 0 1 2 2 2
  spline S112 degree 2 poles (0.1709, 96.3859) (0.0916, 96.3859) (0.0223, 96.4354) knots 0 0 0 1 1 1
  spline S113 degree 2 poles (0.0223, 96.4354) (-0.3308, 96.6895) (-0.7598, 96.6895) knots 0 0 0 1 1 1
  spline S114 degree 2 poles (-0.7598, 96.6895) (-1.0371, 96.6895) (-1.4595, 96.4684) (-1.4595, 96.2704) knots 0 0 0 1 2 2 2
  spline S115 degree 2 poles (-1.4595, 96.2704) (-1.4595, 96.1549) (-1.377, 96.0921) knots 0 0 0 1 1 1
  line L208 (-1.377, 96.0921) -> (0.0817, 94.9304)
  spline S116 degree 2 poles (0.0817, 94.9304) (0.4712, 94.7258) (0.4712, 94.1879) knots 0 0 0 1 1 1
  spline S117 degree 2 poles (0.4712, 94.1879) (0.4712, 93.6235) (-0.3869, 93.1747) (-0.7928, 93.1747) knots 0 0 0 1 2 2 2
  spline S118 degree 2 poles (-0.7928, 93.1747) (-1.3044, 93.1747) (-1.8523, 93.5344) knots 0 0 0 1 1 1
  spline S119 degree 2 poles (-1.8523, 93.5344) (-1.9645, 93.607) (-1.9645, 93.7357) knots 0 0 0 1 1 1
  spline S120 degree 2 poles (-1.9645, 93.7357) (-1.9645, 93.838) (-1.8192, 93.9964) (-1.7136, 93.9964) knots 0 0 0 1 2 2 2
  spline S121 degree 2 poles (-1.7136, 93.9964) (-1.641, 93.9964) (-1.5684, 93.9469) knots 0 0 0 1 1 1
  spline S122 degree 2 poles (-1.5684, 93.9469) (-1.1559, 93.6796) (-0.7862, 93.6796) knots 0 0 0 1 1 1
  spline S123 degree 2 poles (-0.7862, 93.6796) (-0.4991, 93.6796) (-0.2252, 93.8215) knots 0 0 0 1 1 1
  spline S124 degree 2 poles (-0.2252, 93.8215) (-0.0206, 93.9337) (-0.0206, 94.1846) knots 0 0 0 1 1 1
  spline S125 degree 2 poles (-0.0206, 94.1846) (-0.0206, 94.4684) (-0.2285, 94.6235) knots 0 0 0 1 1 1
  line L209 (-0.2285, 94.6235) -> (-1.6839, 95.7852)
  spline S126 degree 2 poles (-1.6839, 95.7852) (-1.948, 95.8941) (-1.948, 96.277) knots 0 0 0 1 1 1
  spline S127 degree 2 poles (-1.948, 96.277) (-1.948, 96.7753) (-1.4892, 97.0162) knots 0 0 0 1 1 1
  spline S128 degree 2 poles (-1.4892, 97.0162) (-1.1658, 97.1813) (-0.7598, 97.1813) knots 0 0 0 1 1 1
  spline S129 degree 2 poles (-0.7598, 97.1813) (-0.1625, 97.1813) (0.3029, 96.8512) knots 0 0 0 1 1 1
  spline S130 degree 2 poles (3.953, 93.4453) (3.953, 93.1945) (3.7022, 93.1945) knots 0 0 0 1 1 1
  spline S131 degree 2 poles (3.7022, 93.1945) (3.4514, 93.1945) (3.4514, 93.4453) knots 0 0 0 1 1 1
  line L210 (3.4514, 93.4453) -> (3.4514, 96.1549)
  line L211 (3.4514, 96.1549) -> (2.7319, 94.8149)
  spline S132 degree 2 poles (2.7319, 94.8149) (2.6659, 94.6961) (2.5372, 94.6961) knots 0 0 0 1 1 1
  spline S133 degree 2 poles (2.5372, 94.6961) (2.4118, 94.6961) (2.3227, 94.8413) knots 0 0 0 1 1 1
  line L212 (2.3227, 94.8413) -> (1.623, 96.1549)
  line L213 (1.623, 96.1549) -> (1.623, 93.4453)
  spline S134 degree 2 poles (1.623, 93.4453) (1.623, 93.1945) (1.3722, 93.1945) knots 0 0 0 1 1 1
  spline S135 degree 2 poles (1.3722, 93.1945) (1.1213, 93.1945) (1.1213, 93.4453) knots 0 0 0 1 1 1
  line L214 (1.1213, 93.4453) -> (1.1213, 96.9139)
  spline S136 degree 2 poles (1.1213, 96.9139) (1.1213, 97.1945) (1.3524, 97.1945) knots 0 0 0 1 1 1
  spline S137 degree 2 poles (1.3524, 97.1945) (1.4976, 97.1945) (1.5966, 96.9568) knots 0 0 0 1 1 1
  line L215 (1.5966, 96.9568) -> (2.5372, 95.409)
  line L216 (2.5372, 95.409) -> (3.4844, 97.0426)
  spline S138 degree 2 poles (3.4844, 97.0426) (3.5735, 97.1945) (3.7154, 97.1945) knots 0 0 0 1 1 1
  spline S139 degree 2 poles (3.7154, 97.1945) (3.953, 97.1945) (3.953, 96.9139) knots 0 0 0 1 1 1
  line L217 (3.953, 96.9139) -> (3.953, 93.4453)
  line L218 (-21.2938, 100.503) -> (-21.8666, 98.7778)
  spline S140 degree 2 poles (-21.8666, 98.7778) (-21.9532, 98.5047) (-22.2263, 98.5047) knots 0 0 0 1 1 1
  spline S141 degree 2 poles (-22.2263, 98.5047) (-22.6393, 98.5047) (-22.6393, 98.8844) knots 0 0 0 1 1 1
  spline S142 degree 2 poles (-22.6393, 98.8844) (-22.6393, 98.9576) (-22.6127, 99.0309) knots 0 0 0 1 1 1
  line L219 (-22.6127, 99.0309) -> (-20.2147, 106.2116)
  spline S143 degree 2 poles (-20.2147, 106.2116) (-20.1014, 106.5513) (-19.8417, 106.5513) knots 0 0 0 1 1 1
  spline S144 degree 2 poles (-19.8417, 106.5513) (-19.5752, 106.5513) (-19.4686, 106.2116) knots 0 0 0 1 1 1
  line L220 (-19.4686, 106.2116) -> (-17.0706, 99.0309)
  spline S145 degree 2 poles (-17.0706, 99.0309) (-17.0507, 98.9576) (-17.0507, 98.8844) knots 0 0 0 1 1 1
  spline S146 degree 2 poles (-17.0507, 98.8844) (-17.0507, 98.5047) (-17.4636, 98.5047) knots 0 0 0 1 1 1
  spline S147 degree 2 poles (-17.4636, 98.5047) (-17.7367, 98.5047) (-17.8233, 98.7778) knots 0 0 0 1 1 1
  line L221 (-17.8233, 98.7778) -> (-18.3962, 100.503)
  line L222 (-18.3962, 100.503) -> (-21.2938, 100.503)
  line L223 (-18.6693, 101.3157) -> (-19.8417, 104.8327)
  line L224 (-19.8417, 104.8327) -> (-21.0207, 101.3157)
  line L225 (-21.0207, 101.3157) -> (-18.6693, 101.3157)
  line L226 (-11.5219, 103.2807) -> (-11.5219, 106.0917)
  spline S148 degree 2 poles (-11.5219, 106.0917) (-11.5219, 106.4914) (-11.1223, 106.4914) knots 0 0 0 1 1 1
  spline S149 degree 2 poles (-11.1223, 106.4914) (-10.7226, 106.4914) (-10.7226, 106.0917) knots 0 0 0 1 1 1
  line L227 (-10.7226, 106.0917) -> (-10.7226, 98.911)
  spline S150 degree 2 poles (-10.7226, 98.911) (-10.7226, 98.5047) (-11.1289, 98.5047) knots 0 0 0 1 1 1
  spline S151 degree 2 poles (-11.1289, 98.5047) (-11.5219, 98.5047) (-11.5219, 98.8977) knots 0 0 0 1 1 1
  line L228 (-11.5219, 98.8977) -> (-11.5219, 102.4814)
  line L229 (-11.5219, 102.4814) -> (-14.7059, 102.4814)
  line L230 (-14.7059, 102.4814) -> (-14.7059, 98.8977)
  spline S152 degree 2 poles (-14.7059, 98.8977) (-14.7059, 98.498) (-15.1056, 98.498) knots 0 0 0 1 1 1
  spline S153 degree 2 poles (-15.1056, 98.498) (-15.5053, 98.498) (-15.5053, 98.8977) knots 0 0 0 1 1 1
  line L231 (-15.5053, 98.8977) -> (-15.5053, 106.0717)
  spline S154 degree 2 poles (-15.5053, 106.0717) (-15.5053, 106.4714) (-15.1056, 106.4714) knots 0 0 0 1 1 1
  spline S155 degree 2 poles (-15.1056, 106.4714) (-14.7059, 106.4714) (-14.7059, 106.0717) knots 0 0 0 1 1 1
  line L232 (-14.7059, 106.0717) -> (-14.7059, 103.2807)
  line L233 (-14.7059, 103.2807) -> (-11.5219, 103.2807)
  line L234 (-7.1256, 105.672) -> (-8.7243, 105.672)
  spline S156 degree 2 poles (-8.7243, 105.672) (-9.1239, 105.672) (-9.1239, 106.0717) knots 0 0 0 1 1 1
  spline S157 degree 2 poles (-9.1239, 106.0717) (-9.1239, 106.4714) (-8.7243, 106.4714) knots 0 0 0 1 1 1
  line L235 (-8.7243, 106.4714) -> (-4.7342, 106.4714)
  spline S158 degree 2 poles (-4.7342, 106.4714) (-4.3346, 106.4714) (-4.3346, 106.0717) knots 0 0 0 1 1 1
  spline S159 degree 2 poles (-4.3346, 106.0717) (-4.3346, 105.672) (-4.7342, 105.672) knots 0 0 0 1 1 1
  line L236 (-4.7342, 105.672) -> (-6.3329, 105.672)
  line L237 (-6.3329, 105.672) -> (-6.3329, 98.8977)
  spline S160 degree 2 poles (-6.3329, 98.8977) (-6.3329, 98.498) (-6.7259, 98.498) knots 0 0 0 1 1 1
  spline S161 degree 2 poles (-6.7259, 98.498) (-7.1256, 98.498) (-7.1256, 98.8977) knots 0 0 0 1 1 1
  line L238 (-7.1256, 98.8977) -> (-7.1256, 105.672)
  line L239 (-1.9366, 103.2807) -> (0.0684, 103.2807)
  spline S162 degree 2 poles (0.0684, 103.2807) (0.4614, 103.2807) (0.4614, 102.881) knots 0 0 0 1 1 1
  spline S163 degree 2 poles (0.4614, 102.881) (0.4614, 102.4814) (0.0684, 102.4814) knots 0 0 0 1 1 1
  line L240 (0.0684, 102.4814) -> (-1.9366, 102.4814)
  line L241 (-1.9366, 102.4814) -> (-1.9366, 99.2974)
  line L242 (-1.9366, 99.2974) -> (0.8611, 99.2974)
  spline S164 degree 2 poles (0.8611, 99.2974) (1.2608, 99.2974) (1.2608, 98.8977) knots 0 0 0 1 1 1
  spline S165 degree 2 poles (1.2608, 98.8977) (1.2608, 98.498) (0.8611, 98.498) knots 0 0 0 1 1 1
  line L243 (0.8611, 98.498) -> (-2.3362, 98.498)
  spline S166 degree 2 poles (-2.3362, 98.498) (-2.7359, 98.498) (-2.7359, 98.871) knots 0 0 0 1 1 1
  line L244 (-2.7359, 98.871) -> (-2.7359, 106.0717)
  spline S167 degree 2 poles (-2.7359, 106.0717) (-2.7359, 106.4714) (-2.3362, 106.4714) knots 0 0 0 1 1 1
  line L245 (-2.3362, 106.4714) -> (0.8611, 106.4714)
  spline S168 degree 2 poles (0.8611, 106.4714) (1.2608, 106.4714) (1.2608, 106.0717) knots 0 0 0 1 1 1
  spline S169 degree 2 poles (1.2608, 106.0717) (1.2608, 105.672) (0.8611, 105.672) knots 0 0 0 1 1 1
  line L246 (0.8611, 105.672) -> (-1.9366, 105.672)
  line L247 (-1.9366, 105.672) -> (-1.9366, 103.2807)
  line L248 (6.8294, 103.2807) -> (6.8294, 106.0917)
  spline S170 degree 2 poles (6.8294, 106.0917) (6.8294, 106.4914) (7.2291, 106.4914) knots 0 0 0 1 1 1
  spline S171 degree 2 poles (7.2291, 106.4914) (7.6288, 106.4914) (7.6288, 106.0917) knots 0 0 0 1 1 1
  line L249 (7.6288, 106.0917) -> (7.6288, 98.911)
  spline S172 degree 2 poles (7.6288, 98.911) (7.6288, 98.5047) (7.2225, 98.5047) knots 0 0 0 1 1 1
  spline S173 degree 2 poles (7.2225, 98.5047) (6.8294, 98.5047) (6.8294, 98.8977) knots 0 0 0 1 1 1
  line L250 (6.8294, 98.8977) -> (6.8294, 102.4814)
  line L251 (6.8294, 102.4814) -> (3.6454, 102.4814)
  line L252 (3.6454, 102.4814) -> (3.6454, 98.8977)
  spline S174 degree 2 poles (3.6454, 98.8977) (3.6454, 98.498) (3.2458, 98.498) knots 0 0 0 1 1 1
  spline S175 degree 2 poles (3.2458, 98.498) (2.8461, 98.498) (2.8461, 98.8977) knots 0 0 0 1 1 1
  line L253 (2.8461, 98.8977) -> (2.8461, 106.0717)
  spline S176 degree 2 poles (2.8461, 106.0717) (2.8461, 106.4714) (3.2458, 106.4714) knots 0 0 0 1 1 1
  spline S177 degree 2 poles (3.2458, 106.4714) (3.6454, 106.4714) (3.6454, 106.0717) knots 0 0 0 1 1 1
  line L254 (3.6454, 106.0717) -> (3.6454, 103.2807)
  line L255 (3.6454, 103.2807) -> (6.8294, 103.2807)
  line L256 (13.2108, 103.2807) -> (13.2108, 106.0917)
  spline S178 degree 2 poles (13.2108, 106.0917) (13.2108, 106.4914) (13.6105, 106.4914) knots 0 0 0 1 1 1
  spline S179 degree 2 poles (13.6105, 106.4914) (14.0101, 106.4914) (14.0101, 106.0917) knots 0 0 0 1 1 1
  line L257 (14.0101, 106.0917) -> (14.0101, 98.911)
  spline S180 degree 2 poles (14.0101, 98.911) (14.0101, 98.5047) (13.6038, 98.5047) knots 0 0 0 1 1 1
  spline S181 degree 2 poles (13.6038, 98.5047) (13.2108, 98.5047) (13.2108, 98.8977) knots 0 0 0 1 1 1
  line L258 (13.2108, 98.8977) -> (13.2108, 102.4814)
  line L259 (13.2108, 102.4814) -> (10.0268, 102.4814)
  line L260 (10.0268, 102.4814) -> (10.0268, 98.8977)
  spline S182 degree 2 poles (10.0268, 98.8977) (10.0268, 98.498) (9.6271, 98.498) knots 0 0 0 1 1 1
  spline S183 degree 2 poles (9.6271, 98.498) (9.2275, 98.498) (9.2275, 98.8977) knots 0 0 0 1 1 1
  line L261 (9.2275, 98.8977) -> (9.2275, 106.0717)
  spline S184 degree 2 poles (9.2275, 106.0717) (9.2275, 106.4714) (9.6271, 106.4714) knots 0 0 0 1 1 1
  spline S185 degree 2 poles (9.6271, 106.4714) (10.0268, 106.4714) (10.0268, 106.0717) knots 0 0 0 1 1 1
  line L262 (10.0268, 106.0717) -> (10.0268, 103.2807)
  line L263 (10.0268, 103.2807) -> (13.2108, 103.2807)
  spline S186 degree 2 poles (19.5921, 100.4897) (19.5921, 99.6637) (18.4265, 98.498) (17.6005, 98.498) knots 0 0 0 1 2 2 2
  line L264 (17.6005, 98.498) -> (16.0085, 98.498)
  spline S187 degree 2 poles (16.0085, 98.498) (15.8486, 98.498) (15.6088, 98.7378) (15.6088, 98.8977) knots 0 0 0 1 2 2 2
  line L265 (15.6088, 98.8977) -> (15.6088, 106.0717)
  spline S188 degree 2 poles (15.6088, 106.0717) (15.6088, 106.4714) (16.0085, 106.4714) knots 0 0 0 1 1 1
  spline S189 degree 2 poles (16.0085, 106.4714) (16.4081, 106.4714) (16.4081, 106.0717) knots 0 0 0 1 1 1
  line L266 (16.4081, 106.0717) -> (16.4081, 103.2807)
  line L267 (16.4081, 103.2807) -> (17.6005, 103.2807)
  spline S190 degree 2 poles (17.6005, 103.2807) (18.4331, 103.2807) (19.5921, 102.115) (19.5921, 101.289) knots 0 0 0 1 2 2 2
  line L268 (19.5921, 101.289) -> (19.5921, 100.4897)
  line L269 (18.7928, 100.4897) -> (18.7928, 101.289)
  spline S191 degree 2 poles (18.7928, 101.289) (18.7928, 101.782) (18.0934, 102.4814) (17.6005, 102.4814) knots 0 0 0 1 2 2 2
  line L270 (17.6005, 102.4814) -> (16.4081, 102.4814)
  line L271 (16.4081, 102.4814) -> (16.4081, 99.2974)
  line L272 (16.4081, 99.2974) -> (17.6005, 99.2974)
  spline S192 degree 2 poles (17.6005, 99.2974) (18.0934, 99.2974) (18.7928, 99.9968) (18.7928, 100.4897) knots 0 0 0 1 2 2 2
  spline S193 degree 2 poles (21.1908, 98.8977) (21.1908, 98.498) (20.7911, 98.498) knots 0 0 0 1 1 1
  spline S194 degree 2 poles (20.7911, 98.498) (20.3915, 98.498) (20.3915, 98.8977) knots 0 0 0 1 1 1
  line L273 (20.3915, 98.8977) -> (20.3915, 106.0717)
  spline S195 degree 2 poles (20.3915, 106.0717) (20.3915, 106.4714) (20.7911, 106.4714) knots 0 0 0 1 1 1
  spline S196 degree 2 poles (20.7911, 106.4714) (21.1908, 106.4714) (21.1908, 106.0717) knots 0 0 0 1 1 1
  line L274 (21.1908, 106.0717) -> (21.1908, 98.8977)
  line L275 (15.6566, 93.1771) -> (14.1087, 93.1771)
  spline S197 degree 2 poles (14.1087, 93.1771) (13.8579, 93.1771) (13.8579, 93.4279) knots 0 0 0 1 1 1
  line L276 (13.8579, 93.4279) -> (13.8579, 96.9131)
  spline S198 degree 2 poles (13.8579, 96.9131) (13.8579, 97.1639) (14.1087, 97.1639) knots 0 0 0 1 1 1
  spline S199 degree 2 poles (14.1087, 97.1639) (14.3595, 97.1639) (14.3595, 96.9131) knots 0 0 0 1 1 1
  line L277 (14.3595, 96.9131) -> (14.3595, 93.6755)
  line L278 (14.3595, 93.6755) -> (15.6566, 93.6755)
  spline S200 degree 2 poles (15.6566, 93.6755) (15.9107, 93.6755) (15.9107, 93.4279) knots 0 0 0 1 1 1
  spline S201 degree 2 poles (15.9107, 93.4279) (15.9107, 93.1771) (15.6566, 93.1771) knots 0 0 0 1 1 1
  spline S202 degree 2 poles (19.013, 94.2035) (19.013, 93.7778) (18.4123, 93.1771) (17.9833, 93.1771) knots 0 0 0 1 2 2 2
  line L279 (17.9833, 93.1771) -> (17.5972, 93.1771)
  spline S203 degree 2 poles (17.5972, 93.1771) (17.1681, 93.1771) (16.5708, 93.7745) (16.5708, 94.2035) knots 0 0 0 1 2 2 2
  line L280 (16.5708, 94.2035) -> (16.5708, 96.1408)
  spline S204 degree 2 poles (16.5708, 96.1408) (16.5708, 96.5633) (17.1681, 97.1639) (17.5972, 97.1639) knots 0 0 0 1 2 2 2
  line L281 (17.5972, 97.1639) -> (17.9833, 97.1639)
  spline S205 degree 2 poles (17.9833, 97.1639) (18.4123, 97.1639) (19.013, 96.56) (19.013, 96.1408) knots 0 0 0 1 2 2 2
  line L282 (19.013, 96.1408) -> (19.013, 94.2035)
  line L283 (18.5114, 94.2002) -> (18.5114, 96.1408)
  spline S206 degree 2 poles (18.5114, 96.1408) (18.5114, 96.3553) (18.2011, 96.6656) (17.9833, 96.6656) knots 0 0 0 1 2 2 2
  line L284 (17.9833, 96.6656) -> (17.5972, 96.6656)
  spline S207 degree 2 poles (17.5972, 96.6656) (17.3793, 96.6656) (17.0724, 96.3586) (17.0724, 96.1408) knots 0 0 0 1 2 2 2
  line L285 (17.0724, 96.1408) -> (17.0724, 94.2002)
  spline S208 degree 2 poles (17.0724, 94.2002) (17.0724, 93.9824) (17.3793, 93.6755) (17.5972, 93.6755) knots 0 0 0 1 2 2 2
  line L286 (17.5972, 93.6755) -> (17.9833, 93.6755)
  spline S209 degree 2 poles (17.9833, 93.6755) (18.2011, 93.6755) (18.5114, 93.9857) (18.5114, 94.2002) knots 0 0 0 1 2 2 2
  spline S210 degree 2 poles (22.1153, 95.9461) (22.1153, 95.5336) (21.6203, 94.8867) (21.277, 94.7976) knots 0 0 0 1 2 2 2
  line L287 (21.277, 94.7976) -> (22.0757, 93.5567)
  spline S211 degree 2 poles (22.0757, 93.5567) (22.1186, 93.4874) (22.1186, 93.4246) knots 0 0 0 1 1 1
  spline S212 degree 2 poles (22.1186, 93.4246) (22.1186, 93.3223) (21.9569, 93.1738) (21.8546, 93.1738) knots 0 0 0 1 2 2 2
  spline S213 degree 2 poles (21.8546, 93.1738) (21.7259, 93.1738) (21.65, 93.2926) knots 0 0 0 1 1 1
  line L288 (21.65, 93.2926) -> (20.7523, 94.7283)
  line L289 (20.7523, 94.7283) -> (20.1747, 94.7283)
  line L290 (20.1747, 94.7283) -> (20.1747, 93.4279)
  spline S214 degree 2 poles (20.1747, 93.4279) (20.1747, 93.1771) (19.9239, 93.1771) knots 0 0 0 1 1 1
  spline S215 degree 2 poles (19.9239, 93.1771) (19.6731, 93.1771) (19.6731, 93.4279) knots 0 0 0 1 1 1
  line L291 (19.6731, 93.4279) -> (19.6731, 96.9131)
  spline S216 degree 2 poles (19.6731, 96.9131) (19.6731, 97.0154) (19.8216, 97.1639) (19.9239, 97.1639) knots 0 0 0 1 2 2 2
  line L292 (19.9239, 97.1639) -> (20.8942, 97.1639)
  spline S217 degree 2 poles (20.8942, 97.1639) (21.3991, 97.1639) (22.1153, 96.4478) (22.1153, 95.9461) knots 0 0 0 1 2 2 2
  spline S218 degree 2 poles (21.6137, 95.9461) (21.6137, 96.2431) (21.1912, 96.6656) (20.8942, 96.6656) knots 0 0 0 1 2 2 2
  line L293 (20.8942, 96.6656) -> (20.1747, 96.6656)
  line L294 (20.1747, 96.6656) -> (20.1747, 95.2266)
  line L295 (20.1747, 95.2266) -> (20.8942, 95.2266)
  spline S219 degree 2 poles (20.8942, 95.2266) (21.1912, 95.2266) (21.6137, 95.6491) (21.6137, 95.9461) knots 0 0 0 1 2 2 2
  line L296 (23.5543, 94.1507) -> (23.277, 93.319)
  spline S220 degree 2 poles (23.277, 93.319) (23.2341, 93.1804) (23.0559, 93.1804) knots 0 0 0 1 1 1
  spline S221 degree 2 poles (23.0559, 93.1804) (22.7985, 93.1804) (22.7985, 93.4213) knots 0 0 0 1 1 1
  spline S222 degree 2 poles (22.7985, 93.4213) (22.7985, 93.4676) (22.815, 93.5105) knots 0 0 0 1 1 1
  line L297 (22.815, 93.5105) -> (23.9932, 97.0319)
  spline S223 degree 2 poles (23.9932, 97.0319) (24.046, 97.2035) (24.2176, 97.2035) knots 0 0 0 1 1 1
  spline S224 degree 2 poles (24.2176, 97.2035) (24.3859, 97.2035) (24.442, 97.0385) knots 0 0 0 1 1 1
  line L298 (24.442, 97.0385) -> (25.617, 93.5105)
  spline S225 degree 2 poles (25.617, 93.5105) (25.6302, 93.4643) (25.6302, 93.4213) knots 0 0 0 1 1 1
  spline S226 degree 2 poles (25.6302, 93.4213) (25.6302, 93.1804) (25.3694, 93.1804) knots 0 0 0 1 1 1
  spline S227 degree 2 poles (25.3694, 93.1804) (25.1978, 93.1804) (25.1516, 93.3223) knots 0 0 0 1 1 1
  line L299 (25.1516, 93.3223) -> (24.8777, 94.1507)
  line L300 (24.8777, 94.1507) -> (23.5543, 94.1507)
  line L301 (24.7292, 94.659) -> (24.2176, 96.2563)
  line L302 (24.2176, 96.2563) -> (23.7028, 94.659)
  line L303 (23.7028, 94.659) -> (24.7292, 94.659)
  line L304 (-21.1876, 73.6489) -> (-21.9632, 73.6489)
  spline S228 degree 2 poles (-21.9632, 73.6489) (-22.389, 73.6489) (-22.9863, 74.2463) (-22.9863, 74.6753) knots 0 0 0 1 2 2 2
  line L305 (-22.9863, 74.6753) -> (-22.9863, 76.6126)